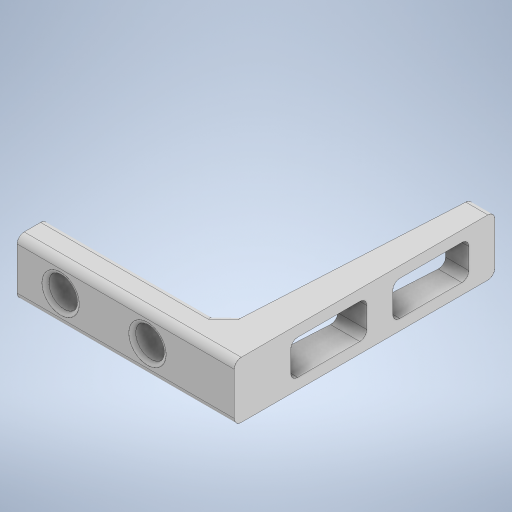
# Autodesk Inventor part: noga1
Saved by Autodesk Inventor 2024.2 (Build 282272000, 272)
## iProperties
Created: 2024-06-19
Part Number: noga1
Material: Ogólny
Document SubType Name: Modeling
Designer: Konrad
Density: 1 g/cm^3
Appearance: Domyślna
Author: Konrad
Autodesk Inventor part; units mm, degrees
ref_plane "YZ Plane" through (0, 0, 0) normal (1, 0, 0) x (0, 1, 0)
ref_plane "XZ Plane" through (0, 0, 0) normal (0, 1, 0) x (-1, 0, 0)
ref_plane "XY Plane" through (0, 0, 0) normal (0, 0, 1) x (1, 0, 0)
sketch "Szkic1" plane through (0, 0, 0) normal (0, 1, 0) x (-1, 0, 0)
  line L0 (0, 0) -> (25, 0)
  line L1 (25, 0) -> (25, -3.5)
  line L2 (25, -3.5) -> (4, -3.5)
  line L3 (4, -3.5) -> (2.5, -30)
  line L4 (2.5, -30) -> (0, -30)
  line L5 (0, -30) -> (0, 0)
  dimension "d0" = 25
  dimension "d1" = 30
  dimension "d2" = 3.5
  dimension "d3" = 2.5
  dimension "d4" = 4
  constraints: 12 end point, 3 perpendicular, 1 horizontal, 1 parallel
  measures "d0" distance of L0.start L0.end
  measures "d1" distance of L4.end L0.start
  measures "d2" distance of L0.end L1.end
  measures "d3" distance of L3.end L4.end
  measures "d4" distance from line of L5 L2.end
extrude "Wyciągnięcie proste1" add sketch "Szkic1" along normal blind 6.5
sketch "Szkic2" plane through (0, 0, 0) normal (1, 0, 0) x (0, 0, -1)
  line L0 (0, 0) -> (30, 0) projected
  line L1 (30, 0) -> (30, 6.5) projected
  line L2 (0, 6.5) -> (30, 6.5) projected
  line L3 (0, 0) -> (0, 6.5) projected
  line L4 (30, 3.25) -> (0, 3.25) construction
  line L5 (18.25, 5.25) -> (27, 5.25)
  line L6 (27, 5.25) -> (27, 1.25)
  line L7 (27, 1.25) -> (18.25, 1.25)
  line L8 (18.25, 1.25) -> (18.25, 5.25)
  line L9 (18.25, 5.25) -> (27, 1.25) construction
  line L10 (27, 5.25) -> (18.25, 1.25) construction
  line L11 (6.5, 5.25) -> (15.25, 5.25)
  line L12 (15.25, 5.25) -> (15.25, 1.25)
  line L13 (15.25, 1.25) -> (6.5, 1.25)
  line L14 (6.5, 1.25) -> (6.5, 5.25)
  line L15 (6.5, 5.25) -> (15.25, 1.25) construction
  line L16 (15.25, 5.25) -> (6.5, 1.25) construction
  line L17 (3.5, 0) -> (3.5, 6.5) projected
  point P0 (22.625, 3.25)
  point P1 (10.875, 3.25)
  dimension "d7" = 26.5
  dimension "d8" = 3
  dimension "d9" = 3
  dimension "d10" = 3
  dimension "d11" = 4
  constraints: 26 end point, 6 midpoint, 4 parallel, 3 point on line, 2 horizontal, 2 perpendicular, 1 collinear
  measures "d7" distance between parallel lines of L1 L17
  measures "d8" distance between parallel lines of L6 L1
  measures "d9" distance between parallel lines of L14 L17
  measures "d10" distance between parallel lines of L8 L12
  measures "d11" distance of L5.end L6.end
extrude "Wyciągnięcie proste2" cut sketch "Szkic2" against normal up to surface contours L5 L6 L7 L8 | L11 L12 L13 L14 surface through (-2.5, 0, -30) normal (-0.9984018, 0, -0.0565133)
sketch "Szkic3" plane through (-25, 0, 0) normal (0, 0, 1) x (1, 0, 0)
  line L0 (0, 0) -> (25, 0) projected
  line L1 (25, 0) -> (25, 6.5) projected
  line L2 (0, 6.5) -> (25, 6.5) construction
  line L3 (0, 0) -> (0, 6.5) projected
  line L4 (0, 3.25) -> (25, 3.25) construction
  circle A0 centre (15, 3.25) radius 1.75
  circle A1 centre (5, 3.25) radius 1.75
  dimension "d14" = 3.5
  dimension "d15" = 10
  dimension "d16" = 10
  constraints: 2 centre point, 2 end point, 2 midpoint, 2 point on line, 1 equal radius
  measures "d14" diameter of A0
  measures "d15" distance from line of L1 A0.centre
  measures "d16" distance of A0.centre A1.centre
extrude "Wyciągnięcie proste3" cut sketch "Szkic3" against normal up to surface (3.5 mm away)
chamfer "Faza1" distance 2 angle 45 1 edges at (-4, 3.25, -3.5)
fillet "Zaokrąglenie1" radius 0.8 16 edges at (-1.25, 6.5, -30) (-1.25, 0, -30) (-12.5, 6.5, 0) (-12.5, 0, 0) (-15.5, 0, -3.5) (-15.5, 6.5, -3.5) (-4.9435, 6.5, -4.4984) (-4.9435, 0, -4.4984) (-1.3349, 5.25, -27) (-1.5825, 5.25, -18.25) (-1.3349, 1.25, -27) (-1.5825, 1.25, -18.25) (-1.6675, 5.25, -15.25) (-1.6675, 1.25, -15.25) (-1.9151, 1.25, -6.5) (-1.9151, 5.25, -6.5)
fillet "Zaokrąglenie2" radius 0.4 4 edges at (-11.75, 3.25, -3.5) (-21.75, 3.25, -3.5) (-11.75, 3.25, 0) (-21.75, 3.25, 0)
equation "\"d9\" = d8"
